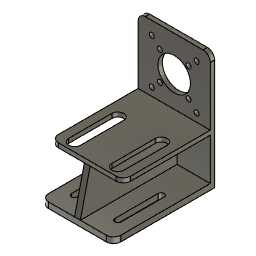
Nema17_5to1_mount v3 (Autodesk Fusion 360 design; units mm, degrees)
Autodesk Fusion 360 part; units mm, degrees
sketch "Sketch1" plane through (0, 0, 0) normal (0, 1, 0) x (1, 0, 0)
  line L0 (0, 0) -> (50, 0)
  line L1 (50, 0) -> (50, -49)
  line L2 (50, -49) -> (0, -49)
  line L3 (0, -49) -> (0, 0)
  line L4 (0, -24.5) -> (50, -24.5) construction
  line L5 (25, -49) -> (25, 0) construction
  circle A0 centre (25, -24.5) radius 11.25
  circle A1 centre (25, -24.5) radius 14 construction
  line L6 (0, -49) -> (0, -40) construction
  line L7 (0, -40) -> (9.5, -40) construction
  circle A2 centre (9.5, -40) radius 1.75
  line L8 (9.5, -40) -> (25, -24.5) construction
  circle A3 centre (15.1005, -34.3995) radius 1.75
  circle A4 centre (40.5, -40) radius 1.75
  circle A5 centre (34.8995, -34.3995) radius 1.75
  circle A6 centre (40.5, -9) radius 1.75
  circle A7 centre (34.8995, -14.6005) radius 1.75
  circle A8 centre (15.1005, -14.6005) radius 1.75
  circle A9 centre (9.5, -9) radius 1.75
  line L9 (0, -49) -> (5, -49)
  line L10 (5, -49) -> (5, -44) construction
  line L11 (5, -44) -> (0, -44) construction
  line L12 (0, -44) -> (0, -49)
  arc A10 (0, -44) -> (5, -49) centre (5, -44) ccw
  arc A11 (45, -49) -> (50, -44) centre (45, -44) ccw
  dimension "d1" = 50
  dimension "d2" = 49
  dimension "d3" = 22.5
  dimension "d4" = 28
  dimension "d5" = 9
  dimension "d6" = 9.5
  dimension "d7" = 3.5
  dimension "d8" = 3.5
  dimension "d11" = 5
  dimension "d12" = 5
  constraint horizontal L0
  constraint vertical L1
  constraint horizontal L2
  constraint vertical L3
  constraint coincident L0.start L3.end
  constraint midpoint L3 L4.start
  constraint midpoint L1 L4.end
  constraint midpoint L2 L5.start
  constraint midpoint L0 L5.end
  constraint midpoint L5 A0.centre
  constraint concentric A0 A1
  constraint perpendicular L2 L6
  constraint perpendicular L6 L7
  constraint coincident L7.end A2.centre
  constraint coincident A0.centre A1.centre
  constraint coincident L8 A3.centre
  constraint coincident A1 A3.centre
  constraint symmetric L5 A2 A4
  constraint symmetric L5 A3 A5
  constraint symmetric L4 A2 A9
  constraint symmetric L4 A3 A8
  constraint symmetric L4 A4 A6
  constraint symmetric L4 A5 A7
  constraint horizontal L9
  constraint vertical L10
  constraint horizontal L11
  constraint vertical L12
  constraint tangent L6 A10
  constraint symmetric L5 L9.end A11.start
  constraint symmetric L5 L11.end A11.end
  constraint symmetric L5 A10 A11
  measures "d1" distance of L0.start L0.end
  measures "d2" distance of L0.start L2.end
  measures "d3" diameter of A0
  measures "d4" diameter of A1
  measures "d5" distance of L2.end L6.end
  measures "d6" distance of L6.end L7.end
  measures "d7" diameter of A2
  measures "d8" diameter of A3
  measures "d11" distance of L2.end L9.end
  measures "d12" distance of L2.end L11.end
extrude "Extrude2" add sketch "Sketch1" along normal blind 3 contours L0 L1 L2 L3 A10 A11
sketch "Sketch2" plane through (0, 0, 0) normal (0, 0, 1) x (1, 0, 0)
  line L0 (0, 3) -> (50, 3)
  line L1 (50, 3) -> (50, -67)
  line L2 (50, -67) -> (0, -67)
  line L3 (0, -67) -> (0, 3)
  line L4 (25, -67) -> (25, 3) construction
  line L5 (0, -67) -> (10, -67) construction
  line L6 (10, -67) -> (10, -54) construction
  line L7 (10, -54) -> (7.9, -54) construction
  line L8 (7.9, -54) -> (12.1, -54)
  line L9 (12.1, -54) -> (12.1, -24)
  line L10 (12.1, -24) -> (7.9, -24)
  line L11 (7.9, -24) -> (7.9, -54)
  arc A0 (7.9, -54) -> (12.1, -54) centre (10, -54) ccw
  arc A1 (12.1, -24) -> (7.9, -24) centre (10, -24) ccw
  arc A2 (37.9, -54) -> (42.1, -54) centre (40, -54) ccw
  line L12 (37.9, -54) -> (37.9, -24)
  line L13 (42.1, -24) -> (42.1, -54)
  arc A3 (42.1, -24) -> (37.9, -24) centre (40, -24) ccw
  line L14 (0, 0) -> (50, 0)
  point P0 (0, 3)
  dimension "d15" = 70
  dimension "d16" = 10
  dimension "d17" = 13
  dimension "d18" = 2.1
  dimension "d19" = 4.2
  dimension "d20" = 30
  constraint horizontal L0
  constraint vertical L1
  constraint horizontal L2
  constraint vertical L3
  constraint coincident P0 L0.start
  constraint midpoint L2 L4.start
  constraint midpoint L0 L4.end
  constraint perpendicular L3 L5
  constraint perpendicular L2 L6
  constraint perpendicular L6 L7
  constraint horizontal L8
  constraint vertical L9
  constraint horizontal L10
  constraint vertical L11
  constraint tangent L9 A0
  constraint tangent L11 A1
  constraint symmetric L4 L7.end A2.end
  constraint symmetric L4 L8.end A2.start
  constraint symmetric L4 L9.end L12.end
  constraint symmetric L4 L10.end L13.start
  constraint symmetric L4 A0 A2
  constraint symmetric L4 A1 A3
  constraint coincident L14.start origin
  constraint coincident L1 L14.end
  constraint perpendicular L1 L14
  measures "d15" distance of P0 L2.end
  measures "d16" distance of L2.end L5.end
  measures "d17" distance of L5.end L6.end
  measures "d18" distance of L6.end L7.end
  measures "d19" distance of L7.end L8.end
  measures "d20" distance of L7.end L10.end
extrude "Extrude6" add sketch "Sketch2" against normal blind 32.6
extrude "Extrude7" cut sketch "Sketch2" against normal blind 28.6 contours L1 L2 L3 L14
ref_plane "WorkPlane1" through (25, -32, 5.7) normal (1, 0, 0) x (0, 0, -1)
sketch "Sketch6" plane through (25, -32, 5.7) normal (1, 0, 0) x (0, 1, 0)
  line L0 (32, -34.3) -> (-35, -34.3)
  line L1 (-35, -34.3) -> (-35, -5.3)
  line L2 (-35, -5.3) -> (32, -5.3)
  line L3 (32, -5.3) -> (32, -34.3)
  point P0 (32, -34.3)
  dimension "d48" = 67
  dimension "d49" = 29
  constraint horizontal L0
  constraint vertical L1
  constraint horizontal L2
  constraint vertical L3
  constraint coincident P0 L0.start
  measures "d48" distance of P0 L0.end
  measures "d49" distance of P0 L2.end
sketch "Sketch10" plane through (0, 0, 0) normal (0, -1, 0) x (1, 0, 0)
  circle A0 centre (25, 24.5) radius 11.25
  circle A1 centre (9.5, 40) radius 1.75
  circle A2 centre (40.5, 40) radius 1.75
  circle A3 centre (15.1005, 34.3995) radius 1.75
  circle A4 centre (34.8995, 34.3995) radius 1.75
  circle A5 centre (40.5, 9) radius 1.75
  circle A6 centre (34.8995, 14.6005) radius 1.75
  circle A7 centre (15.1005, 14.6005) radius 1.75
  circle A8 centre (9.5, 9) radius 1.75
  arc A9 (5, 49) -> (0, 44) centre (5, 44) ccw
  line L0 (0, 44) -> (0, -28.6)
  line L1 (0, -28.6) -> (50, -28.6)
  line L2 (50, -28.6) -> (50, 44)
  arc A10 (50, 44) -> (45, 49) centre (45, 44) ccw
  line L3 (45, 49) -> (5, 49)
  line L4 (25, 24.5) -> (25, 3.4) construction
  dimension "d71" = 21.1
  constraint coincident A0.centre L4.start
  constraint vertical L4
  measures "d71" distance of A0.centre L4.end
extrude "Extrude15" add sketch "Sketch6" along normal blind 2 and the other way blind 2
sketch "Sketch11" plane through (0, 0, 0.4) normal (0, 0, 1) x (-1, 0, 0)
  line L0 (-23, 67) -> (-27, 67)
  line L1 (-27, 67) -> (-27, 0)
  line L2 (-27, 0) -> (-23, 0)
  line L3 (-23, 0) -> (-23, 67)
  line L4 (0, 0) -> (-50, 0)
  line L5 (-50, 0) -> (-50, 60.1926)
  line L6 (-50, 60.1926) -> (0, 60.1926)
  line L7 (0, 60.1926) -> (0, 0)
  line L8 (-50, -3) -> (-50, 67)
  line L9 (-7.9, 24) -> (-5.9, 24)
  line L10 (-5.9, 24) -> (-14.1, 24)
  line L11 (-14.1, 24) -> (-14.1, 54)
  line L12 (-14.1, 54) -> (-5.9, 54)
  line L13 (-5.9, 54) -> (-5.9, 24)
  arc A0 (-5.9, 54) -> (-14.1, 54) centre (-10, 54) ccw
  arc A1 (-14.1, 24) -> (-5.9, 24) centre (-10, 24) ccw
  line L14 (-25, 67) -> (-25, 0)
  line L15 (-25, 60.1926) -> (-25, 53.1429)
  line L16 (-35.9, 24) -> (-35.9, 54)
  line L17 (-44.1, 54) -> (-44.1, 24)
  arc A2 (-35.9, 54) -> (-44.1, 54) centre (-40, 54) ccw
  arc A3 (-44.1, 24) -> (-35.9, 24) centre (-40, 24) ccw
  point P0 (-7.9, 24)
  dimension "d76" = 2
  dimension "d77" = 8.2
  constraint horizontal L4
  constraint vertical L5
  constraint horizontal L6
  constraint vertical L7
  constraint coincident L5.end L8
  constraint coincident L4.start L7.end
  constraint coincident P0 L9.start
  constraint horizontal L9
  constraint horizontal L10
  constraint vertical L11
  constraint horizontal L12
  constraint vertical L13
  constraint tangent L13 A1
  constraint midpoint L6 L15.start
  constraint coincident L14 L15.end
  constraint perpendicular L6 L15
  constraint symmetric L9.end L14 L17.end
  constraint symmetric L10.end L14 L16.start
  constraint symmetric L11.end L14 L16.end
  constraint symmetric L12.end L14 L17.start
  constraint symmetric A0 L14 A2
  constraint symmetric A1 L14 A3
  measures "d76" distance of P0 L9.end
  measures "d77" distance of L9.end L10.end
extrude "Extrude16" add sketch "Sketch11" along normal blind 3 contours L3 L4 L6 L7 | L2 L3 L4 L6 L14 L15 | L1 L2 L4 L6 L14 L15 | L1 L4 L5 L6 L8
sketch "Sketch12" plane through (27, 0, 0) normal (1, 0, 0) x (0, 1, 0)
  line L0 (0, 0.4) -> (-60.1926, 0.4)
  line L1 (-60.1926, 0.4) -> (-67, 0.4)
  line L2 (-67, 0.4) -> (-67, -28.6)
  line L3 (-67, -28.6) -> (0, -28.6)
  line L4 (0, -28.6) -> (0, 0.4)
  line L5 (-60.1926, 0.4) -> (-67, -28.6)
  line L6 (-67, 0.4) -> (-60.1926, 0.4)
  constraint coincident L0.end L1.start
  constraint coincident L2.end L3.start
  constraint coincident L1.end L2.start
extrude "Extrude17" cut sketch "Sketch12" against normal blind 8 contours L1 L2 L5 L6
fillet "Fillet3" radius 5 4 edges at (0, -60.1926, 1.9) (0, -67, -30.6) (50, -67, -30.6) (50, -60.1926, 1.9)
